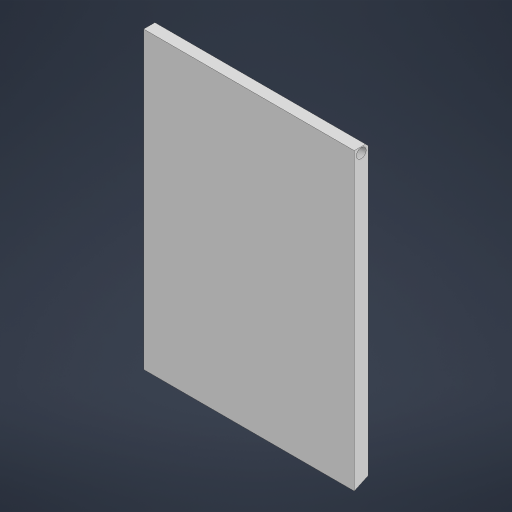
# Autodesk Inventor part: stojka - správná verze
Saved by Autodesk Inventor 2024 (Build 280153000, 153)
## iProperties
Created: 2024-01-22
Part Number: stojka - správná verze
Material: Generic
Document SubType Name: Modeling
Designer: Tomáš
Density: 1 g/cm^3
Appearance: Default
Author: Tomáš
Autodesk Inventor part; units mm, degrees
ref_plane "YZ Plane" through (0, 0, 0) normal (1, 0, 0) x (0, 1, 0)
ref_plane "XZ Plane" through (0, 0, 0) normal (0, 1, 0) x (-1, 0, 0)
ref_plane "XY Plane" through (0, 0, 0) normal (0, 0, 1) x (1, 0, 0)
sketch "Sketch1" plane through (0, 0, 0) normal (0, 0, 1) x (1, 0, 0)
  line L0 (0, 0) -> (75, 0)
  line L1 (75, 0) -> (75, -105)
  line L2 (75, -105) -> (0, -105)
  line L3 (0, -105) -> (0, 0)
  dimension "d0" = 75
  dimension "d1" = 105
  constraints: 8 end point, 2 parallel, 1 horizontal, 1 perpendicular
  measures "d0" distance of L1.end L2.end
  measures "d1" distance of L0.end L1.end
extrude "Extrusion1" add sketch "Sketch1" along normal blind 5
sketch "Sketch2" plane through (75, -105, 0) normal (1, 0, 0) x (0, 0, -1)
  line L0 (-5, 0) -> (-5, 105) projected
  line L1 (0, 0) -> (0, 105) projected
  line L2 (-5, 105) -> (0, 105)
  line L3 (0, 105) -> (0, 102)
  line L4 (0, 102) -> (-5, 102)
  line L5 (-5, 102) -> (-5, 105)
  circle A0 centre (-2.5, 103) radius 1.75
  line L6 (0, 105) -> (-1, 105)
  line L7 (0, 105) -> (-5, 105) projected
  line L8 (0, 105) -> (0, 104)
  line L9 (-1, 105) -> (0, 104)
  point P0 (-1, 105)
  point P1 (0, 104)
  point P2 (-2.5, 105)
  point P3 (-2.5, 105)
  dimension "d4" = 3
  dimension "d5" = 3.5
  dimension "d6" = 1
  dimension "d7" = 1
  dimension "d14" = 2
  constraints: 14 end point, 3 point on line, 2 midpoint, 2 parallel, 1 centre point, 1 horizontal, 1 perpendicular, 1 vertical alignment
  measures "d4" distance of L2.end L3.end
  measures "d5" diameter of A0
  measures "d6" distance of L2.end L6.end
  measures "d7" distance of L2.end L8.end
  measures "d14" distance of point (-2.5, 105) A0.centre
extrude "Extrusion2" cut sketch "Sketch2" against normal through all contours A0 L4 | L4 A0
extrude "Extrusion3" cut sketch "Sketch2" against normal through all contours L2 L1 L9
sketch "Sketch3" plane through (75, -105, 5) normal (1, 0, 0) x (0, 0, -1)
  line L0 (0, 105) -> (0, 0) projected
  line L1 (5, 104) -> (5, 0) projected
  line L2 (0, 0) -> (5, 2.3157)
  line L3 (5, 0) -> (5, 104) projected
  line L4 (5, 0) -> (0, 0) projected
  line L5 (5, 2.3157) -> (5, 0)
  line L6 (5, 0) -> (0, 0)
  point P0 (5, 105)
  constraints: 6 end point, 1 perpendicular, 1 point on line, 1 vertical
extrude "Extrusion4" cut sketch "Sketch3" against normal through all
body "Solid1"
